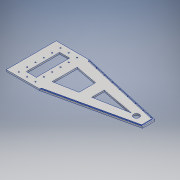
# Autodesk Inventor part: W1sup
Saved by Autodesk Inventor 2017 (Build 210142000, 142)
## iProperties
Created: 2016-12-01
Part Number: W1sup
Material: Aluminum 6061
Document SubType Name: Sheet Metal
Designer: aesen
Density: 2.7 g/cm^3
Sheet Metal Rule: Default_mm
Appearance: Aluminum - Flat
Author: aesen
Autodesk Inventor part; units mm, degrees
ref_plane "YZ Plane" through (0, 0, 0) normal (1, 0, 0) x (0, 1, 0)
ref_plane "XZ Plane" through (0, 0, 0) normal (0, 1, 0) x (-1, 0, 0)
sketch "Sketch1" plane through (0, 0, 0) normal (0, 0, 1) x (1, 0, 0)
  line L0 (-400, -150.0109) -> (-400, 0)
  circle A0 centre (-350, -125) radius 3.5
  circle A1 centre (-300, -125) radius 3.5
  circle A2 centre (-250, -125) radius 3.5
  circle A3 centre (-350, -75) radius 3.5
  circle A4 centre (-250, -75) radius 3.5
  circle A5 centre (-350, -25) radius 3.5
  circle A6 centre (-250, -25) radius 3.5
  line L1 (-330, -100) -> (-270, -100)
  line L2 (-270, -100) -> (-270, 0)
  line L3 (-330, 0) -> (-330, -100)
  line L4 (293.2796, -30.0061) -> (-199.5823, -140.5264)
  line L5 (-199.5608, -75) -> (200.421, -0.0307)
  line L6 (299.6046, -34.9531) -> (-199.5823, -146.9202)
  line L7 (-199.5588, -150.0109) -> (305.238, -36.7909)
  line L8 (-400, -150.0109) -> (-199.5588, -150.0109)
  circle A7 centre (-139.6396, -130.2873) radius 3.5
  circle A8 centre (-79.6396, -116.8294) radius 3.5
  circle A9 centre (-19.6396, -103.3714) radius 3.5
  circle A10 centre (40.3604, -89.9135) radius 3.5
  circle A11 centre (100.3828, -76.4523) radius 3.5
  circle A12 centre (160.3828, -62.9943) radius 3.5
  circle A13 centre (220.3828, -49.5364) radius 3.5
  circle A14 centre (280.3828, -36.0784) radius 3.5
  line L9 (0.4301, -37.5154) -> (0.4301, -0.0319)
  line L10 (-63.836, -49.5609) -> (-63.836, -0.0245)
  line L11 (-199.5823, -146.9202) -> (-199.5823, -140.5264)
  line L12 (-199.5608, -75) -> (-199.5608, 0)
  arc A15 (214.4084, 0) -> (249.3334, 0) centre (231.8709, 0) ccw
  line L13 (293.2796, 0) -> (293.2796, -30.0061)
  line L14 (299.6046, 0) -> (299.6046, -9.3443)
  line L15 (299.6046, -9.3443) -> (299.6046, -34.9531)
  line L16 (305.238, 0) -> (305.238, -36.7909)
  line L17 (293.2796, 30.0061) -> (-199.5823, 140.5264)
  line L18 (-199.5608, 74.934) -> (200.421, -0.0307)
  circle A16 centre (-300, 125) radius 3.5
  circle A17 centre (-250, 125) radius 3.5
  circle A18 centre (-350, 125) radius 3.5
  circle A19 centre (-250, 25) radius 3.5
  line L19 (-270, 100) -> (-270, 0)
  circle A20 centre (-350, 25) radius 3.5
  line L20 (-330, 100) -> (-270, 100)
  circle A21 centre (-350, 75) radius 3.5
  line L21 (-330, 0) -> (-330, 100)
  line L22 (-400, 150.0109) -> (-400, 0)
  circle A22 centre (-250, 75) radius 3.5
  line L23 (299.6046, 34.9531) -> (-199.5823, 146.9202)
  line L24 (-199.5588, 150.0109) -> (305.238, 36.7909)
  line L25 (-400, 150.0109) -> (-199.5588, 150.0109)
  circle A23 centre (-139.6396, 130.2873) radius 3.5
  circle A24 centre (-79.6396, 116.8294) radius 3.5
  circle A25 centre (-19.6396, 103.3714) radius 3.5
  circle A26 centre (40.3604, 89.9135) radius 3.5
  circle A27 centre (100.3828, 76.4523) radius 3.5
  circle A28 centre (160.3828, 62.9943) radius 3.5
  circle A29 centre (220.3828, 49.5364) radius 3.5
  circle A30 centre (280.3828, 36.0784) radius 3.5
  line L26 (0.4301, 37.4516) -> (0.4301, -0.0319)
  line L27 (-63.8167, 49.4928) -> (-63.836, -0.0245)
  line L28 (-199.5823, 146.9202) -> (-199.5823, 140.5264)
  line L29 (-199.5608, 74.934) -> (-199.5608, 0)
  arc A31 (249.3334, 0) -> (214.4084, 0) centre (231.8709, 0) ccw
  line L30 (293.2796, 0) -> (293.2796, 30.0061)
  line L31 (299.6046, 0) -> (299.6046, 9.3443)
  line L32 (299.6046, 9.3443) -> (299.6046, 34.9531)
  line L33 (305.238, 0) -> (305.238, 36.7909)
  circle A32 centre (296.4421, 17.9624) radius 3.5
  circle A33 centre (296.4421, -18.0376) radius 3.5
  point P0 (0, 0)
  point P1 (297.0951, -0.0376)
  constraints: 68 end point, 34 centre point, 5 vertical, 4 point on circle, 2 midpoint, 2 point on line, 1 horizontal
sketch "Sketch17" plane through (0, 0, 0) normal (0, 0, 1) x (1, 0, 0)
  line L0 (293.2796, -30.0061) -> (-199.5823, -140.5264)
  line L1 (299.6046, -34.9531) -> (-199.5823, -146.9202)
  line L2 (-199.5823, -146.9202) -> (-199.5823, -140.5264)
  line L3 (293.2796, 0) -> (293.2796, -30.0061)
  line L4 (299.6046, 0) -> (299.6046, -9.3443)
  line L5 (299.6046, -9.3443) -> (299.6046, -34.9531)
  line L6 (293.2796, 30.0061) -> (-199.5823, 140.5264)
  line L7 (293.2796, 0) -> (293.2796, 30.0061)
  line L8 (299.6046, 9.3443) -> (299.6046, 34.9531)
  line L9 (299.6046, 34.9531) -> (-199.5823, 146.9202)
  line L10 (299.6046, 0) -> (299.6046, 9.3443)
  line L11 (-199.5823, 146.9202) -> (-199.5823, 140.5264)
  constraints: 24 end point, 3 vertical
sketch "Sketch16" plane through (0, 0, 0) normal (0, 0, 1) x (1, 0, 0)
  circle A0 centre (-139.6396, -130.2873) radius 3.5
  circle A1 centre (-79.6396, -116.8294) radius 3.5
  circle A2 centre (-19.6396, -103.3714) radius 3.5
  circle A3 centre (40.3604, -89.9135) radius 3.5
  circle A4 centre (100.3828, -76.4523) radius 3.5
  circle A5 centre (160.3828, -62.9943) radius 3.5
  circle A6 centre (220.3828, -49.5364) radius 3.5
  circle A7 centre (280.3828, -36.0784) radius 3.5
  circle A8 centre (280.3828, 36.0784) radius 3.5
  circle A9 centre (220.3828, 49.5364) radius 3.5
  circle A10 centre (160.3828, 62.9943) radius 3.5
  circle A11 centre (100.3828, 76.4523) radius 3.5
  circle A12 centre (40.3604, 89.9135) radius 3.5
  circle A13 centre (-139.6396, 130.2873) radius 3.5
  circle A14 centre (-79.6396, 116.8294) radius 3.5
  circle A15 centre (-19.6396, 103.3714) radius 3.5
  circle A16 centre (296.4421, 17.9624) radius 3.5
  circle A17 centre (296.4421, -18.0376) radius 3.5
  constraints: 18 centre point
extrude "Extrusion12" add sketch "Sketch1" along normal blind 9.525 contours L0 L22 L25 L24 L33 L16 L7 L8 | L13 A33 L15 L6 A14 L4 | A14 L6 L4 | L4 A14 | A33 L13 | L13 A33 L15 | A14 L6 A13 L4 | L13 L30 A32 L32 L31 L14 L15 A33 | L15 A33 | A13 L6 L4 | L4 A13 | L6 A14 | A13 L6 A12 L4 | A13 L6 | A32 L30 | L30 A32 L32 | A12 L6 L4 | L4 A12 | L30 L17 A30 L23 L32 A32 | L32 A32 | A12 L6 A11 L4 | A12 L6 | A11 L6 L4 | L4 A11 | A30 L17 | L17 A30 L23 | A11 L6 A10 L4 | A11 L6 | L17 A29 L23 A30 | L23 A30 | A10 L6 L4 | L4 A10 | A29 L17 | L17 A29 L23 | A10 L6 A9 L4 | A10 L6 | L17 A28 L23 A29 | L23 A29 | A9 L6 L4 | L4 A9 | A28 L17 | L17 A28 L23 | A9 L6 A8 L4 | A9 L6 | L17 A27 L23 A28 | L23 A28 | A8 L6 L4 | L4 A8 | A27 L17 | L17 A27 L23 | A8 L6 A7 L4 | A8 L6 | L17 A26 L23 A27 | L23 A27 | A7 L6 L4 | L4 A7 | A26 L17 | L17 A26 L23 | A7 L6 L11 L4 | A7 L6 | L17 A25 L23 A26 | L23 A26 | A25 L17 | L17 A25 L23 | L17 A24 L23 A25 | L23 A25 | A24 L17 | L17 A24 L23 | L17 A23 L23 A24 | L23 A24 | A23 L17 | L17 A23 L23 | L17 L28 L23 A23 | L23 A23 | L10 L27 L18 L26 L9 L5
hole "Hole15" at (-139.6396, -130.2873, 0) at (-79.6396, -116.8294, 0) at (-19.6396, -103.3714, 0) at (40.3604, -89.9135, 0) at (100.3828, -76.4523, 0) at (160.3828, -62.9943, 0) at (220.3828, -49.5364, 0) at (280.3828, -36.0784, 0) at (296.4421, 17.9624, 0) at (296.4421, -18.0376, 0) at (280.3828, 36.0784, 0) at (220.3828, 49.5364, 0) at (160.3828, 62.9943, 0) at (100.3828, 76.4523, 0) at (40.3604, 89.9135, 0) at (-19.6396, 103.3714, 0) at (-79.6396, 116.8294, 0) at (-139.6396, 130.2873, 0) direction (0, 0, 1) diameter 4.978 end through all countersink diameter 7 countersink angle 90 thread size "1/4-20 UNC" class "2B" standard "ANSI Unified Screw Threads"
ref_plane "Work Plane13" through (-400, 150.0109, 9.525) normal (0, 0, -1) x (0, -1, 0)
sketch "Sketch19" plane through (0, 0, 9.525) normal (0, 0, 1) x (1, 0, 0)
  line L0 (293.2796, -30.0061) -> (-199.5823, -140.5264)
  line L1 (299.6046, -34.9531) -> (-199.5823, -146.9202)
  line L2 (-199.5823, -146.9202) -> (-199.5823, -140.5264)
  line L3 (293.2796, 0) -> (293.2796, -30.0061)
  line L4 (299.6046, 0) -> (299.6046, -9.3443)
  line L5 (299.6046, -9.3443) -> (299.6046, -34.9531)
  line L6 (293.2796, 30.0061) -> (-199.5823, 140.5264)
  line L7 (293.2796, 0) -> (293.2796, 30.0061)
  line L8 (299.6046, 9.3443) -> (299.6046, 34.9531)
  line L9 (299.6046, 34.9531) -> (-199.5823, 146.9202)
  line L10 (299.6046, 0) -> (299.6046, 9.3443)
  line L11 (-199.5823, 146.9202) -> (-199.5823, 140.5264)
  point P0 (0, 0)
  constraints: 24 end point, 3 vertical
emboss "Emboss9" sketch "Sketch19" operation cut depth 3 direction (0, 0, -1)
equation "\"BendRadius\" = Thickness"
equation "\"BendReliefWidth\" = Thickness"
equation "\"BendReliefDepth\" = 0.5 * Thickness"
equation "\"CornerReliefSize\" = 4 * Thickness"
equation "\"MinimumRemnant\" = 2 * Thickness"
equation "\"TransitionRadius\" = BendRadius"
equation "\"JacobiRadiusSize\" = BendRadius"
equation "\"GapSize\" = Thickness"
equation "\"Thickness\" = 0.5"
body "Solid11"
